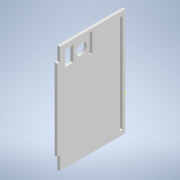
# Autodesk Inventor part: divider
Saved by Autodesk Inventor 2022 (Build 260153070, 153G)
## iProperties
Created: 2022-05-12
Part Number: divider
Material: Generic
Document SubType Name: Modeling
Designer: Jeanette Guo
Density: 1 g/cm^3
Appearance: Default
Author: Jeanette Guo
Autodesk Inventor part; units mm, degrees
ref_plane "YZ Plane" through (0, 0, 0) normal (1, 0, 0) x (0, 1, 0)
ref_plane "XZ Plane" through (0, 0, 0) normal (0, 1, 0) x (-1, 0, 0)
ref_plane "XY Plane" through (0, 0, 0) normal (0, 0, 1) x (1, 0, 0)
sketch "Sketch1" plane through (0, 0, 0) normal (0, 0, 1) x (1, 0, 0)
  line L0 (-56.5, -25) -> (-59.5, -25) projected
  line L1 (-59.5, -25) -> (-59.5, 65) projected
  line L2 (-56.5, -38) -> (-56.5, 78) projected
  line L3 (-59.5, 65) -> (-56.5, 65) projected
  line L4 (-56.5, -25) -> (-59.5, -25)
  line L5 (-59.5, -25) -> (-59.5, 65)
  line L6 (-59.5, 65) -> (-56.5, 65)
  line L7 (-56.5, 65) -> (-56.5, -25)
  point P0 (0, 0)
  constraints: 8 end point, 2 parallel, 1 horizontal, 1 perpendicular
extrude "Extrusion1" add sketch "Sketch1" along normal blind 76
sketch "Sketch2" plane through (-59.5, -25, 0) normal (0, -1, 0) x (1, 0, 0)
  line L0 (3, 0) -> (3, 76) projected
  line L1 (0, 76) -> (3, 76) projected
  line L2 (3, 0) -> (0, 0)
  line L3 (0, 0) -> (0, 76)
  line L4 (0, 76) -> (3, 76)
  line L5 (3, 76) -> (3, 0)
  point P0 (59.5, 0)
  constraints: 8 end point, 2 parallel, 1 horizontal, 1 perpendicular
extrude "Extrusion2" add sketch "Sketch2" along normal blind 13.5
sketch "Sketch4" plane through (-59.5, 65, 0) normal (0, 1, 0) x (1, 0, 0)
  line L0 (3, 0) -> (3, -76) projected
  line L1 (3, 0) -> (0, 0) projected
  line L2 (3, -76) -> (0, -76)
  line L3 (0, -76) -> (0, 0)
  line L4 (0, 0) -> (3, 0)
  line L5 (3, 0) -> (3, -76)
  point P0 (59.5, 0)
  constraints: 8 end point, 2 parallel, 1 horizontal, 1 perpendicular
extrude "Extrusion3" add sketch "Sketch4" along normal blind 16.5
sketch "Sketch5" plane through (-59.5, -38.5, 0) normal (-1, 0, 0) x (0, 0, 1)
  line L0 (0, 120) -> (76, 120) projected
  line L1 (76, 120) -> (73, 120)
  line L2 (73, 120) -> (73, 110)
  line L3 (73, 110) -> (76, 110)
  line L4 (76, 110) -> (76, 120)
  line L5 (76, 0) -> (76, 120) projected
  line L6 (76, 0) -> (73, 0)
  line L7 (73, 0) -> (73, 10)
  line L8 (73, 10) -> (76, 10)
  line L9 (76, 10) -> (76, 0)
  point P0 (0, 38.5)
  dimension "d10" = 3
  dimension "d11" = 10
  dimension "d12" = 3
  dimension "d13" = 10
  constraints: 16 end point, 4 parallel, 2 horizontal, 2 perpendicular
  measures "d10" distance of L3.end L2.end
  measures "d11" distance of L2.end L1.end
  measures "d12" distance of L7.end L8.end
  measures "d13" distance of L6.end L7.end
extrude "Extrusion4" cut sketch "Sketch5" against normal blind 10
sketch "Sketch6" plane through (0, 0, 76) normal (0, 0, 1) x (1, 0, 0)
  line L0 (-59.5, -28.5) -> (-56.5, -28.5) projected
  line L1 (-56.5, -28.5) -> (-56.5, -38.5) projected
  line L2 (-59.5, -38.5) -> (-59.5, -28.5) projected
  line L3 (-56.5, -23.5) -> (-59.5, -23.5) projected
  line L4 (-59.5, 66.5) -> (-56.5, 66.5) projected
  line L5 (-59.5, 81.5) -> (-59.5, -38.5) projected
  line L6 (-56.5, -23.5) -> (-59.5, -23.5)
  line L7 (-59.5, -23.5) -> (-59.5, -38.5)
  line L8 (-59.5, -38.5) -> (-56.5, -38.5)
  line L9 (-56.5, -38.5) -> (-56.5, -23.5)
  line L10 (-56.5, 66.5) -> (-59.5, 66.5)
  line L11 (-59.5, 66.5) -> (-59.5, 81.5)
  line L12 (-59.5, 81.5) -> (-56.5, 81.5)
  line L13 (-56.5, 81.5) -> (-56.5, 66.5)
  point P0 (0, 0)
  dimension "d16" = 15
  constraints: 16 end point, 4 parallel, 2 horizontal, 2 perpendicular, 1 point on line
  measures "d16" distance of L10.end L11.end
extrude "Extrusion5" cut sketch "Sketch6" against normal blind 3
sketch "Sketch7" plane through (-56.5, -38.5, 0) normal (1, 0, 0) x (0, 0, -1)
  circle A0 centre (-58, 105) radius 5 projected
  circle A1 centre (-58, 105) radius 5 projected
  line L0 (-70, 94.5) -> (-43, 94.5)
  line L1 (-43, 94.5) -> (-43, 117.0005)
  line L2 (-43, 117.0005) -> (-70, 117.0005)
  line L3 (-70, 117.0005) -> (-70, 94.5)
  line L4 (0, 91.5) -> (-73, 91.5) projected
  line L5 (-73, 105) -> (-73, 95) projected
  line L6 (-63, 120.0005) -> (-73, 120.0005) projected
  line L7 (-40, 95) -> (-40, 117) projected
  line L8 (-58.25, 97.2505) -> (-58.25, 114.2505) projected
  line L9 (-58.25, 114.2505) -> (-58.25, 97.2505) projected
  line L10 (-58.25, 97.2505) -> (-67.25, 97.2505) projected
  line L11 (-67.25, 97.2505) -> (-67.25, 114.2505) projected
  line L12 (-67.25, 114.2505) -> (-58.25, 114.2505) projected
  line L13 (-58.25, 114.2505) -> (-67.25, 114.2505)
  line L14 (-67.25, 114.2505) -> (-67.25, 97.2505)
  line L15 (-67.25, 97.2505) -> (-58.25, 97.2505)
  line L16 (-58.25, 97.2505) -> (-58.25, 114.2505)
  circle A2 centre (-49.0313, 105.75) radius 6
  line L17 (-73, 120) -> (0, 120) projected
  point P0 (0, 38.5)
  point P1 (-58.25, 100.0063)
  point P2 (-58.25, 109.9937)
  dimension "d26" = 3
  dimension "d27" = 3
  dimension "d28" = 3
  dimension "d29" = 3
  dimension "d30" = 12
  dimension "d31" = 9
  dimension "d32" = 14.25
  dimension "d33" = 14.25
  constraints: 16 end point, 4 parallel, 2 horizontal, 2 perpendicular, 1 centre point
  measures "d26" distance between parallel lines of L4 L0
  measures "d27" distance between parallel lines of L6 L2
  measures "d28" distance between parallel lines of L7 L1
  measures "d29" distance between parallel lines of L3 L5
  measures "d30" diameter of A2
  measures "d31" distance of A1.centre A2.centre
  measures "d32" distance from line of A2.centre L4
  measures "d33" distance from line of L17 A2.centre
extrude "Extrusion6" cut sketch "Sketch7" against normal blind 3 contours A0 A2 | A0 A2 | L8 A0 | A0 L8 L10 L11 L12
sketch "Sketch8" plane through (-59.5, -38.5, 0) normal (-1, 0, 0) x (0, 0, 1)
  line L0 (40, 117) -> (40, 95) projected
  line L1 (37, 95) -> (37, 117) projected
  line L2 (37, 117) -> (40, 117) projected
  line L3 (37, 117) -> (40, 117)
  line L4 (40, 117) -> (40, 95)
  line L5 (40, 95) -> (37, 95)
  line L6 (37, 95) -> (37, 117)
  point P0 (0, 38.5)
  point P1 (37, 95)
  constraints: 8 end point, 2 parallel, 1 horizontal, 1 perpendicular
extrude "Extrusion7" cut sketch "Sketch8" against normal blind 3
sketch "Sketch9" plane through (-56.5, -38.5, 0) normal (1, 0, 0) x (0, 0, -1)
  line L0 (-6, 115) -> (-6, 5) projected
  line L1 (-3, 5) -> (-3, 115) projected
  line L2 (-3, 115) -> (-6, 115) projected
  line L3 (-6, 5) -> (-3, 5) projected
  line L4 (-6, 115) -> (-3, 115)
  line L5 (-3, 115) -> (-3, 5)
  line L6 (-3, 5) -> (-6, 5)
  line L7 (-6, 5) -> (-6, 115)
  point P0 (0, 38.5)
  constraints: 8 end point, 2 parallel, 1 horizontal, 1 perpendicular
extrude "Extrusion8" cut sketch "Sketch9" against normal blind 3
sketch "Sketch10" plane through (-56.5, -38.5, 0) normal (1, 0, 0) x (0, 0, -1)
  point P0 (0, 38.5)
body "Solid1"
